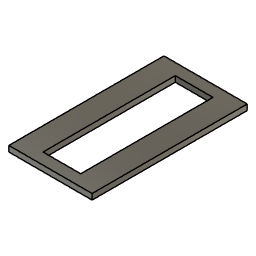
Skirt Holder v1 (Autodesk Fusion 360 design; units mm, degrees)
Autodesk Fusion 360 part; units mm, degrees
sketch "Sketch1" plane through (0, 0, 0) normal (0, 0, 1) x (1, 0, 0)
  line L0 (0, 0) -> (73.04, 0)
  line L1 (0, 0) -> (0, 136.01)
  line L2 (73.04, 136.01) -> (0, 136.01)
  line L3 (73.04, 136.01) -> (73.04, 0)
  line L4 (20, 126.01) -> (53.04, 126.01)
  line L5 (53.04, 126.01) -> (53.04, 10)
  line L6 (20, 126.01) -> (20, 10)
  line L7 (20, 10) -> (53.04, 10)
  dimension "d1" = 73.04
  dimension "d2" = 136.01
  dimension "d4" = 33.04
  dimension "d5" = 116.01
  constraint coincident L0.start L1.start
  constraint horizontal L0
  constraint perpendicular L0 L1
  constraint perpendicular L1 L2
  constraint perpendicular L0 L3
  constraint perpendicular L4 L5
  constraint perpendicular L4 L6
  constraint perpendicular L5 L7
  measures "d1" distance of L0.start L0.end
  measures "d2" distance of L0.start L1.end
  measures "d4" distance of L4.start L4.end
  measures "d5" distance of L4.end L5.end
extrude "Extrude1" add sketch "Sketch1" along normal blind 5
